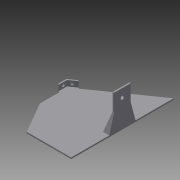
# Autodesk Inventor part: Right Chest
Saved by Autodesk Inventor 2014 SP2 (Build 180246200, 246)
## iProperties
Created: 2015-08-01
Part Number: Right Chest
Material: Generic
Document SubType Name: Modeling
Designer: Devon
Density: 1 g/cm^3
Appearance: Default
Author: Devon
Autodesk Inventor part; units mm, degrees
ref_plane "YZ Plane" through (0, 0, 0) normal (1, 0, 0) x (0, 1, 0)
ref_plane "XZ Plane" through (0, 0, 0) normal (0, 1, 0) x (-1, 0, 0)
ref_plane "XY Plane" through (0, 0, 0) normal (0, 0, 1) x (1, 0, 0)
sketch "Sketch1" plane through (0, 0, 0) normal (0, 1, 0) x (-1, 0, 0)
  line L0 (-24.4733, 28.5935) -> (-24.4733, -206.3565)
  line L1 (-24.4733, -206.3565) -> (118.5711, -106.1957)
  line L2 (-24.4733, -206.3565) -> (150.1517, -206.3565) construction
  line L3 (118.5711, -106.1957) -> (118.5711, -42.6957)
  line L4 (118.5711, -42.6957) -> (77.4122, 28.5935)
  line L5 (-24.4733, 28.5935) -> (77.4122, 28.5935)
  point P0 (0, 0)
  dimension "d0" = 234.95
  dimension "d1" = 174.625
  dimension "d2" = 35
  dimension "d3" = 63.5
  dimension "d4" = 150
  constraints: 12 end point, 2 perpendicular, 1 equal length, 1 horizontal, 1 vertical
  measures "d0" distance of L0.start L0.end
  measures "d1" distance of L0.end L1.end
  measures "d2" angle of L2 L1
  measures "d3" distance of L1.end L3.end
  measures "d4" angle of L4 L3
extrude "Extrusion1" add sketch "Sketch1" along normal blind 3.175
sketch "Sketch2" plane through (0, 3.175, 0) normal (0, 1, 0) x (1, 0, 0)
  line L0 (-77.4122, -28.5935) -> (24.4733, -28.5935) projected
  line L1 (24.4733, -28.5935) -> (24.4733, 206.3565)
  line L2 (21.2983, 88.8815) -> (21.2983, 107.9315)
  line L3 (21.2983, 107.9315) -> (24.4733, 107.9315)
  line L4 (21.2983, 88.8815) -> (21.2983, 69.8315)
  line L5 (21.2983, 69.8315) -> (24.4733, 69.8315)
  point P0 (0, 0)
  dimension "d8" = 19.05
  dimension "d9" = 19.05
  constraints: 10 end point, 2 perpendicular, 2 point on line
  measures "d8" distance of L2.start L2.end
  measures "d9" distance of L2.start L4.end
extrude "Extrusion2" add sketch "Sketch2" along normal blind 79.2734
sketch "Sketch3" plane through (24.4733, 0, 28.5935) normal (1, 0, 0) x (0, 0, -1)
  line L0 (136.525, 82.4484) -> (117.475, 82.4484)
  line L1 (117.475, 82.4484) -> (117.475, 63.3984)
  line L2 (117.475, 63.3984) -> (136.525, 63.3984)
  line L3 (136.525, 63.3984) -> (136.525, 82.4484)
  point P0 (28.5935, 0)
  dimension "d12" = 19.05
  dimension "d13" = 19.05
  constraints: 8 end point, 2 parallel, 1 horizontal, 1 perpendicular
  measures "d12" distance of L2.end L1.end
  measures "d13" distance of L1.end L0.end
hole "Hole1" at (24.4733, 63.3984, -88.8815) direction (-1, 0, 0) diameter 8.3312 end through all
sketch "Sketch4" plane through (0, 3.175, 0) normal (0, 1, 0) x (1, 0, 0)
  line L0 (-102.9662, 117.1224) -> (-118.5711, 106.1957)
  line L1 (-118.5711, 87.1457) -> (-118.5711, 106.1957)
  line L2 (-124.1966, 109.1242) -> (-108.5917, 120.0508)
  line L3 (-124.1966, 109.1242) -> (-124.1966, 90.0742)
  line L4 (-102.9662, 117.1224) -> (-108.5917, 120.0508)
  line L5 (-118.5711, 87.1457) -> (-124.1966, 90.0742)
  point P0 (0, 0)
  dimension "d21" = 19.05
  dimension "d23" = 19.05
  constraints: 12 end point, 3 parallel, 1 point on line
  measures "d21" distance of L1.end L0.start
  measures "d23" distance of L1.end L1.start
extrude "Extrusion3" add sketch "Sketch4" against normal blind 3.175
sketch "Sketch5" plane through (0, 3.175, 0) normal (0, 1, 0) x (1, 0, 0)
  line L0 (-108.5917, 120.0508) -> (-102.9662, 117.1224) projected
  line L1 (-124.1966, 109.1242) -> (-108.5917, 120.0508) projected
  line L2 (-124.1966, 90.0742) -> (-124.1966, 109.1242) projected
  line L3 (-118.5711, 87.1457) -> (-124.1966, 90.0742) projected
  line L4 (-124.1966, 90.0742) -> (-124.1966, 109.1242)
  line L5 (-124.1966, 109.1242) -> (-108.5917, 120.0508)
  line L6 (-108.5917, 120.0508) -> (-105.7755, 118.5848)
  line L7 (-105.7755, 118.5848) -> (-121.3838, 107.6557)
  line L8 (-121.3838, 107.6557) -> (-121.3838, 88.61)
  line L9 (-121.3838, 88.61) -> (-124.1966, 90.0742)
  point P0 (0, 0)
  dimension "d28" = 3.175
  constraints: 12 end point, 3 collinear, 1 midpoint, 1 parallel, 1 point on line
  measures "d28" distance of L0.start L6.end
extrude "Extrusion4" add sketch "Sketch5" along normal blind 12.7
sketch "Sketch6" plane through (-108.5917, 0, -120.0508) normal (-0.5735764, 0, -0.819152) x (-0.819152, 0, 0.5735764)
  line L0 (19.05, 15.875) -> (19.05, 0) projected
  line L1 (0, 15.875) -> (19.05, 15.875)
  line L2 (9.525, 15.875) -> (9.525, 9.525)
  point P0 (-20.0948, 0)
  dimension "d31" = 6.35
  constraints: 4 end point, 2 perpendicular, 1 midpoint
  measures "d31" distance of L2.start L2.end
hole "Hole2" at (-116.3942, 9.525, -114.5875) direction (0.5735764, 0, 0.819152) diameter 6.35 end through all
sketch "Sketch7" plane through (-124.1966, 0, -109.1242) normal (-1, 0, 0) x (0, 0, 1)
  line L0 (0, 15.875) -> (19.05, 15.875) projected
  line L1 (9.525, 15.875) -> (9.525, 9.525)
  point P0 (109.1242, 0)
  dimension "d39" = 6.35
  constraints: 2 end point, 1 midpoint, 1 perpendicular
  measures "d39" distance of L1.start L1.end
hole "Hole3" at (-124.1966, 9.525, -99.5992) direction (1, 0, 0) diameter 6.35 depth 25.4 tip angle 118
sketch "Sketch8" plane through (21.2983, 3.175, -107.9315) normal (-1, 0, 0) x (0, 0, 1)
  line L0 (38.1, 0) -> (0, 0) projected
  line L1 (38.1, 0) -> (38.1, 79.2734) projected
  line L2 (0, 0) -> (0, 79.2734) projected
  line L3 (0, 41.1734) -> (38.1, 41.1734)
  line L4 (38.1, 41.1734) -> (38.1, 0)
  line L5 (38.1, 0) -> (0, 0)
  line L6 (0, 0) -> (0, 41.1734)
  point P0 (107.9315, -3.175)
  dimension "d47" = 38.1
  constraints: 8 end point, 3 perpendicular, 2 point on line, 1 collinear
  measures "d47" distance of L2.end L3.start
extrude "Extrusion5" add sketch "Sketch8" along normal blind 25.4
sketch "Sketch9" plane through (21.2983, 82.4484, -69.8315) normal (0, 0, 1) x (1, 0, 0)
  line L0 (-25.4, -38.1) -> (3.175, -38.1)
  line L1 (3.175, -38.1) -> (3.175, -79.2734)
  line L2 (3.175, -79.2734) -> (-25.4, -79.2734)
  line L3 (-25.4, -79.2734) -> (-25.4, -38.1)
  point P0 (-21.2983, -82.4484)
  constraints: 8 end point, 2 parallel, 1 horizontal, 1 perpendicular
extrude "Extrusion6" add sketch "Sketch9" along normal blind 25.4
sketch "Sketch13" plane through (24.4733, 0, 28.5935) normal (1, 0, 0) x (0, 0, -1)
  line L0 (98.425, 44.3484) -> (98.425, 82.4484) projected
  line L1 (147.5486, 3.175) -> (136.525, 44.3484)
  line L2 (147.5486, 3.175) -> (161.925, 3.175)
  line L3 (136.525, 44.3484) -> (161.925, 44.3484)
  line L4 (161.925, 44.3484) -> (161.925, 3.175)
  point P0 (28.5935, 0)
  constraints: 8 end point, 2 perpendicular, 1 parallel
split_face "Split3"
sketch "Sketch14" plane through (24.4733, 0, 28.5935) normal (1, 0, 0) x (0, 0, -1)
  line L0 (161.925, 3.175) -> (234.95, 3.175) projected
  line L1 (136.525, 3.175) -> (147.5486, 3.175) projected
  line L2 (136.525, 44.3484) -> (136.525, 3.175)
  line L3 (136.525, 3.175) -> (147.5486, 3.175)
  line L4 (147.5486, 3.175) -> (136.525, 44.3484)
  point P0 (28.5935, 0)
  dimension "d73" = 11.0236
  constraints: 6 end point, 1 collinear, 1 perpendicular
  measures "d73" distance of L1.start L1.end
extrude "Extrusion8" add sketch "Sketch14" against normal blind 19.05
sketch "Sketch15" plane through (21.2983, 82.4484, -44.4315) normal (0, 0, 1) x (1, 0, 0)
  line L0 (0, -38.1) -> (-11.1125, -79.2734)
  line L1 (-11.1125, -79.2734) -> (-25.4, -79.2734)
  line L2 (-25.4, -79.2734) -> (-25.4, -38.1)
  line L3 (-25.4, -38.1) -> (0, -38.1)
  point P0 (-21.2983, -82.4484)
  constraints: 8 end point
split body "Split4" sketch "Sketch15" result one side removed curves L0 L1 L2 L3 removed pieces at (13.4073, 17.0298, -77.7394)
sketch "Sketch16" plane through (24.4733, 0, 28.5935) normal (1, 0, 0) x (0, 0, -1)
  line L0 (87.4014, 3.175) -> (98.425, 44.3484)
  line L1 (87.4014, 3.175) -> (73.025, 3.175)
  line L2 (73.025, 3.175) -> (73.025, 44.3484)
  line L3 (73.025, 44.3484) -> (98.425, 44.3484)
  point P0 (28.5935, 0)
  constraints: 8 end point, 2 perpendicular
split body "Split5" sketch "Sketch16" result one side removed curves L3 L0 L1 L2 removed pieces at (18.0769, 30.4936, -57.6903)
body "Solid1"
